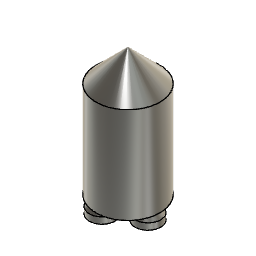
Rocket_like (Autodesk Fusion 360 design; units mm, degrees)
Autodesk Fusion 360 part; units mm, degrees
cylinder "CylinderPrimitive1" add diameter 10 height 20 placed x (1, 0, 0) y (0, 1, 0) z (0, 0, 1) at (0, 0, 0) makes body 1
chamfer "Chamfer1" distance 5 angle 45 1 edges at (-4.6616, -1.8081, 20) on bodies 1
cylinder "CylinderPrimitive2" add diameter 4 height 3 placed x (1, 0, 0) y (0, 1, 0) z (0, 0, 1) at (-9, -14, 0) separate body makes body 2
chamfer "Chamfer2" distance 2 angle 45 1 edges at (-10.8647, -14.7232, 3) on bodies 2
move_body "Move1" bodies 2 to x (1, 0, 0) y (0, 1, 0) z (0, 0, 1) at (5.8279, 18.8439, 0)
move_body "Move2" bodies 2 to x (1, 0, 0) y (0, 1, 0) z (0, 0, 1) at (6.1671, -4.7274, 0)
move_body "Move3" bodies 2 to x (1, 0, 0) y (0, 1, 0) z (0, 0, 1) at (0, 0, -2)
pattern_circular "C-Pattern1" count 3 over 360 about axis through (0, 0, 15) along (0, 0, 1) of bodies 2 makes body 3 at (-1.723, 4.1975, -0.6667) makes body 4 at (-3.0632, -2.652, -0.6667)
component "Base" placed x (1, 0, 0) y (0, 1, 0) z (0, 0, 1) at (0, 0, 0)
